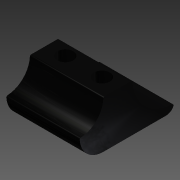
# Autodesk Inventor part: Zawias
Saved by Autodesk Inventor 2015 (Build 190159000, 159)
## iProperties
Created: 2015-12-05
Part Number: Zawias
Material: Stal nierdzewna
Document SubType Name: Modeling
Designer: graaapsik
Density: 8.08 g/cm^3
Appearance: Gładkie - czarne
Mass: 66.1329 g
Surface Area: 41.3842 cm^2
Volume: 8.18476 cm^3
Author: graaapsik
Autodesk Inventor part; units mm, degrees
ref_plane "YZ Plane" through (0, 0, 0) normal (1, 0, 0) x (0, 1, 0)
ref_plane "XZ Plane" through (0, 0, 0) normal (0, 1, 0) x (-1, 0, 0)
ref_plane "XY Plane" through (0, 0, 0) normal (0, 0, 1) x (1, 0, 0)
sketch "Szkic1" plane through (0, 0, 0) normal (0, 0, 1) x (1, 0, 0)
  line L0 (-14, 18) -> (14, 18)
  line L1 (14, 18) -> (14, -18)
  line L2 (14, -18) -> (-14, -18)
  line L3 (-14, -18) -> (-14, 18)
  line L4 (-14, 18) -> (14, -18) construction
  line L5 (14, 18) -> (-14, -18) construction
  point P0 (0, 0)
  dimension "d0" = 28
  dimension "d1" = 36
  constraints: 12 end point, 2 midpoint, 2 parallel, 1 horizontal, 1 perpendicular
  measures "d0" distance of L1.end L2.end
  measures "d1" distance of L0.end L1.end
extrude "Wyciągnięcie proste1" add sketch "Szkic1" along normal mid plane 18
sketch "Szkic3" plane through (0, 0, 0) normal (1, 0, 0) x (0, 1, 0)
  line L0 (-18, 9) -> (-18, -9) construction
  line L1 (-18, 9) -> (18, 9) construction
  line L2 (18, 9) -> (18, -9) construction
  circle A0 centre (-18, 9) radius 9
  circle A1 centre (18, 9.5) radius 16
  point P0 (0, 0)
  dimension "d4" = 18
  dimension "d6" = 32
  dimension "d7" = 0.5
  constraints: 2 centre point, 1 coincident, 1 point on line
  measures "d4" diameter of A0
  measures "d6" diameter of A1
  measures "d7" distance from line of L1 A1.centre
extrude "Wyciągnięcie proste2" cut sketch "Szkic3" along normal mid plane 28
fillet "Zaokrąglenie1" radius 3 1 edges at (0, 18, -9)
fillet "Zaokrąglenie2" radius 9 1 edges at (0, -18, -9)
fillet "Zaokrąglenie3" radius 0.5 5 edges at (0, -9, 9) (0, 2.0078, 9) (0, -18, -0.0001) (0, -18, 0) (0, 18, -6.5)
sketch "Szkic4" plane through (0, 0, -9) normal (0, 0, -1) x (-1, 0, 0)
  line L0 (14, -9) -> (-14, -9) projected
  line L1 (14, -9) -> (14, 15.042) projected
  line L2 (-14, 15.042) -> (14, 15.042) projected
  line L3 (-14, 15.042) -> (-14, -9) projected
  line L4 (-14, 2.0294) -> (14, 2.0294) projected
  line L5 (14, -9.0125) -> (-14, -9.0125) projected
  line L6 (0, 0) -> (0, 3.9534) construction
  point P0 (-7, -2.4906)
  point P1 (7, -2.4906)
  point P2 (-12.5, 2.0294)
  point P3 (12.5, 2.0294)
  point P4 (12.5, -7.0104)
  point P5 (-12.5, -7.0104)
  dimension "d14" = 4.52
  dimension "d15" = 14
  constraints: 2 end point, 1 coincident, 1 symmetric about line, 1 vertical, 1 other
  measures "d14" distance from line of point (-7, -2.491) L4
  measures "d15" distance of point (7, -2.491) point (-7, -2.491)
hole "Otwór1" at (7, -2.4906, -9) at (-7, -2.4906, -9) direction (0, 0, 1) diameter 6 end through all counterbore diameter 11.5 counterbore depth 8
